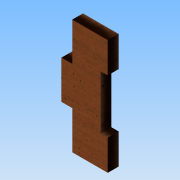
# Autodesk Inventor part: bottom_renfort
Saved by Autodesk Inventor 2015 (Build 190159000, 159)
## iProperties
Created: 2015-12-28
Part Number: bottom_renfort
Material: Générique
Document SubType Name: Modeling
Designer: Gregwar
Density: 1 g/cm^3
Appearance: Par défaut
Author: Gregwar
Autodesk Inventor part; units mm, degrees
ref_plane "YZ Plane" through (0, 0, 0) normal (1, 0, 0) x (0, 1, 0)
ref_plane "XZ Plane" through (0, 0, 0) normal (0, 1, 0) x (-1, 0, 0)
ref_plane "XY Plane" through (0, 0, 0) normal (0, 0, 1) x (1, 0, 0)
sketch "Esquisse1" plane through (0, 0, 0) normal (0, 1, 0) x (-1, 0, 0)
  line L0 (0, 0) -> (9.9, 0)
  line L1 (9.9, 0) -> (9.9, -32)
  line L2 (9.9, -32) -> (0, -32)
  line L3 (0, -32) -> (0, 0)
  line L4 (12.9, -21.3333) -> (9.9, -21.3333)
  line L5 (9.9, -21.3333) -> (9.9, -10.6667)
  line L6 (9.9, -10.6667) -> (12.9, -10.6667)
  line L7 (12.9, -10.6667) -> (12.9, -21.3333)
  point P0 (9.9, -16)
  dimension "d0" = 32
  dimension "d1" = 9.9
  dimension "d2" = 10.6667
  dimension "d3" = 3
  constraints: 16 end point, 4 parallel, 2 horizontal, 2 midpoint, 2 perpendicular
  measures "d0" distance of L2.end L0.start
  measures "d1" distance of L0.start L0.end
  measures "d2" distance of L6.end L4.start
  measures "d3" distance of L4.start L4.end
extrude "Extrusion1" add sketch "Esquisse1" along normal blind 3
sketch "Esquisse2" plane through (0, 3, 0) normal (0, 1, 0) x (1, 0, 0)
  line L0 (-2, 8.5) -> (0, 8.5)
  line L1 (0, 8.5) -> (0, 23.5)
  line L2 (0, 23.5) -> (-2, 23.5)
  line L3 (-2, 23.5) -> (-2, 8.5)
  line L4 (-9.9, 21.3333) -> (-12.9, 21.3333) projected
  line L5 (-12.9, 21.3333) -> (-12.9, 10.6667) projected
  line L6 (-12.9, 10.6667) -> (-9.9, 10.6667) projected
  line L7 (-9.9, 10.6667) -> (-9.9, 0) projected
  line L8 (-9.9, 0) -> (0, 0) projected
  line L9 (0, 0) -> (0, 32) projected
  line L10 (0, 32) -> (-9.9, 32) projected
  line L11 (-9.9, 32) -> (-9.9, 21.3333) projected
  point P0 (0, 16)
  dimension "d6" = 2
  dimension "d7" = 15
  constraints: 8 end point, 2 midpoint, 2 parallel, 1 horizontal, 1 perpendicular
  measures "d6" distance of L1.end L2.end
  measures "d7" distance of L2.end L0.start
extrude "Extrusion2" cut sketch "Esquisse2" against normal through all contours L3 L2 L1 L0
equation "\"d2\" = 0.333333 * d0"
